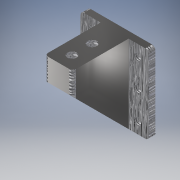
# Autodesk Inventor part: LoadCell_NewBase
Saved by Autodesk Inventor 2019 (Build 230136000, 136)
## iProperties
Created: 2021-04-08
Part Number: LoadCell_NewBase
Material: Aluminum 7075
Document SubType Name: Modeling
Designer: rtavi
Density: 2.81 g/cm^3
Appearance: Satin - Brushed Heavy
Mass: 200.269 g
Surface Area: 192.975 cm^2
Volume: 71.2701 cm^3
Author: rtavi
Autodesk Inventor part; units mm, degrees
ref_plane "YZ Plane" through (0, 0, 0) normal (1, 0, 0) x (0, 1, 0)
ref_plane "XZ Plane" through (0, 0, 0) normal (0, 1, 0) x (-1, 0, 0)
ref_plane "XY Plane" through (0, 0, 0) normal (0, 0, 1) x (1, 0, 0)
sketch "Sketch1" plane through (0, 0, 0) normal (1, 0, 0) x (0, 1, 0)
  line L0 (0, 0) -> (0, 15.4021) construction
  line L1 (-80, 0) -> (0, 0) construction
  line L2 (-10, 16) -> (-10, 44) construction
  line L3 (-10, 56) -> (-10, 0)
  line L4 (-10, 0) -> (-80, 0)
  line L5 (-80, 0) -> (-80, 6)
  line L6 (-80, 6) -> (-30, 56)
  line L7 (-30, 56) -> (-10, 56)
  point P0 (-10, 28)
  dimension "d0" = 6
  dimension "d1" = 70
  dimension "d2" = 56
  dimension "d3" = 20
  constraints: 14 end point, 2 perpendicular, 2 point on line, 2 vertical, 1 horizontal, 1 midpoint, 1 parallel
  measures "d0" distance of L1.start L5.end
  measures "d1" distance between parallel lines of L3 L5
  measures "d2" distance of L3.start L3.end
  measures "d3" distance of L6.end L3.start
extrude "Extrusion1" add sketch "Sketch1" along normal mid plane 25
sketch "Sketch2" plane through (-12.5, -10, 56) normal (0, 1, 0) x (1, 0, 0)
  circle A0 centre (12.5, 12) radius 4.1 construction
  circle A1 centre (12.5, 30) radius 4.1 construction
  point P0 (12.5, 56)
hole "Hole1" at (0, -10, 44) at (0, -10, 26) direction (0, -1, 0) diameter 8.2 depth 16
sketch "Sketch3" plane through (-12.5, -80, 0) normal (0, -1, 0) x (1, 0, 0)
  circle A0 centre (12.5, 44) radius 4.1 construction
  circle A1 centre (12.5, 26) radius 4.1 construction
  point P0 (12.5, 0)
hole "Hole2" at (0, -80, 44) at (0, -80, 26) direction (0, 1, 0) diameter 14 depth 54
sketch "Sketch4" plane through (0, 0, 0) normal (0, 0, 1) x (1, 0, 0)
  line L0 (-30.5, -10) -> (30.5, -10)
  line L1 (30.5, -10) -> (30.5, -30)
  line L2 (30.5, -80) -> (-30.5, -80)
  line L3 (-30.5, -80) -> (-30.5, -60)
  line L4 (0, 0) -> (0, -133.7428) construction
  line L5 (-30.5, -30) -> (-12.5, -30) construction
  line L6 (-12.5, -30) -> (-12.5, -60) construction
  line L7 (-12.5, -10) -> (-12.5, -80) construction
  line L8 (-30.5, -60) -> (-12.5, -60) construction
  line L9 (30.5, -30) -> (12.5, -30) construction
  line L10 (12.5, -80) -> (12.5, -10) construction
  line L11 (12.5, -60) -> (30.5, -60) construction
  line L12 (12.5, -30) -> (12.5, -60) construction
  line L13 (-30.5, -60) -> (-30.5, -30)
  line L14 (30.5, -30) -> (30.5, -60)
  line L15 (30.5, -60) -> (30.5, -80)
  line L16 (-30.5, -30) -> (-30.5, -10)
  dimension "d20" = 30.5
  dimension "d36" = 20
  dimension "d37" = 20
  constraints: 30 end point, 10 parallel, 7 perpendicular, 7 point on line, 3 collinear, 3 horizontal, 1 vertical, 1 other
  measures "d20" distance between parallel lines of L4 L3
  measures "d36" distance between parallel lines of L5 L0
  measures "d37" distance between parallel lines of L8 L2
extrude "Extrusion2" add sketch "Sketch4" along normal blind 6
sketch "Sketch5" plane through (0, 0, 6) normal (0, 0, 1) x (1, 0, 0)
  line L0 (-30.5, -10) -> (30.5, -10) construction
  line L1 (20.5, -10) -> (20.5, -80) construction
  line L2 (30.5, -80) -> (-30.5, -80) construction
  line L3 (30.5, -80) -> (30.5, -10) construction
  line L4 (0, 0) -> (0, -101.1083) construction
  line L5 (12.5, -30) -> (12.5, -80) construction
  line L6 (12.5, -80) -> (30.5, -80)
  point P0 (20.5, -20)
  point P1 (20.5, -70)
  point P2 (-20.5, -20)
  point P3 (-20.5, -70)
  point P4 (20.5, -45)
  point P5 (-20.5, -45)
  dimension "d24" = 10
  dimension "d35" = 50
  dimension "d50" = 25
  dimension "d53" = 10
  constraints: 6 end point, 4 point on line, 3 symmetric about line, 2 vertical, 1 midpoint, 1 perpendicular
  measures "d24" distance from line of L0 point (20.5, -20)
  measures "d35" distance of point (20.5, -70) point (20.5, -20)
  measures "d50" distance of point (20.5, -20) point (20.5, -45)
  measures "d53" distance between parallel lines of L3 L1
hole "Hole3" at (-20.5, -70, 6) at (-20.5, -20, 6) at (20.5, -20, 6) at (20.5, -70, 6) at (-20.5, -45, 6) at (20.5, -45, 6) direction (0, 0, -1) diameter 6.2 end through all
fillet "Fillet1" radius 3 4 edges at (-30.5, -80, 3) (30.5, -80, 3) (30.5, -10, 3) (-30.5, -10, 3)
fillet "Fillet2" radius 3 2 edges at (-12.5, -20, 56) (12.5, -20, 56)
body "Solid1"
